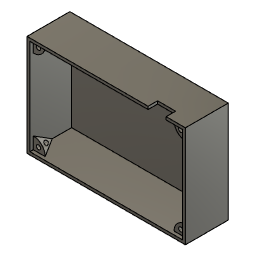
CR_R3 (Autodesk Fusion 360 design; units mm, degrees)
Autodesk Fusion 360 part; units mm, degrees
note: some values were not read from the file. Set by a fixed rule: which sketch regions a step uses.
sketch "Sketch1" plane through (0, 0, 0) normal (0, 0, 1) x (1, 0, 0)
  line L0 (1.5, 1.5) -> (82, 1.5)
  line L1 (82, 1.5) -> (82, 51.9)
  line L2 (82, 51.9) -> (1.5, 51.9)
  line L3 (1.5, 51.9) -> (1.5, 1.5)
  line L4 (83.5, 53.4) -> (0, 53.4)
  line L5 (0, 53.4) -> (0, 0)
  line L6 (0, 0) -> (83.5, 0)
  line L7 (83.5, 0) -> (83.5, 53.4)
  dimension "d6" = 50.4
  dimension "d8" = 1.5
  dimension "d112" = 80.5
  constraint horizontal L0
  constraint vertical L1
  constraint horizontal L2
  constraint vertical L3
  constraint coincident L5.end L6.start
  measures "d6" distance of L0.end L1.end
  measures "d112" distance of L1.end L2.end
extrude "Extrude2" add sketch "Sketch1" along normal blind 1 contours L0 L1 L2 L3
extrude "Extrude3" add sketch "Sketch1" along normal blind 23
sketch "Sketch4" plane through (0, 53.4, 0) normal (0, 1, 0) x (-1, 0, 0)
  line L0 (-83.5, 0) -> (0, 0)
  line L1 (0, 0) -> (0, 23)
  line L2 (0, 23) -> (-83.5, 23)
  line L3 (-83.5, 23) -> (-83.5, 0)
  line L4 (-63.8, 23) -> (-73.3, 23)
  line L5 (-63.8, 18) -> (-73.3, 18)
  line L6 (-73.3, 18) -> (-73.3, 23)
  line L7 (-63.8, 18) -> (-63.8, 23)
  dimension "d49" = 9.5
  dimension "d51" = 9.5
  dimension "d52" = 5
  dimension "d114" = 10.2
  constraint coincident L2 L4.start
  constraint coincident L2 L4.end
  constraint perpendicular L4 L6
  measures "d49" distance of L4.start L4.end
  measures "d51" distance of L5.start L5.end
  measures "d52" distance of L4 L5
  measures "d114" distance of L3 L6
extrude "Extrude8" cut sketch "Sketch4" against normal blind 1.5 contours L2 L4 L5 L6 L7
sketch "Sketch11" plane through (0, 51.9, 0) normal (0, -1, 0) x (1, 0, 0)
  line L0 (63.8, 23) -> (1.5, 23)
  line L1 (1.5, 23) -> (1.5, 1)
  line L2 (1.5, 1) -> (82, 1)
  line L3 (82, 1) -> (82, 23)
  line L4 (1.5, 21.2) -> (7.8, 21.2)
  line L5 (1.5, 21.2) -> (1.5, 11.2)
  line L6 (1.5, 11.2) -> (7.8, 21.2)
  line L7 (82, 21.2) -> (75.7, 21.2)
  line L8 (63.8, 18) -> (63.8, 23)
  line L9 (73.3, 18) -> (63.8, 18)
  line L10 (73.3, 23) -> (73.3, 18)
  line L11 (82, 23) -> (73.3, 23)
  line L12 (82, 21.2) -> (82, 11.2)
  line L13 (82, 11.2) -> (75.7, 21.2)
  dimension "d66" = 6.3
  dimension "d67" = 10
  dimension "d69" = 1.8
  dimension "d79" = 6.3
  dimension "d81" = 1.8
  dimension "d117" = 10
  constraint coincident L1 L4.start
  constraint perpendicular L1 L4
  constraint perpendicular L4 L5
  constraint coincident L3 L7.start
  constraint perpendicular L3 L7
  constraint perpendicular L7 L12
  measures "d66" distance of L4.start L4.end
  measures "d67" distance of L4.start L5.end
  measures "d69" distance of L0.end L4.start
  measures "d79" distance of L7.start L7.end
  measures "d81" distance of L3.end L7.start
  measures "d117" distance of L7.start L12.end
revolve "Revolve1" add sketch "Sketch11" angle 90 about axis through (1.5, 51.9, 21.2) along (0, 0, -1) contours L1 L4 L5 L6
sketch "Sketch12" plane through (0, 0, 21.2) normal (0, 0, 1) x (1, 0, 0)
  arc A0 (1.5, 45.6) -> (7.8, 51.9) centre (1.5, 51.9) ccw
  circle A1 centre (4.25, 49.4) radius 1.125
  line L0 (7.8, 51.9) -> (1.5, 51.9)
  line L1 (1.5, 51.9) -> (1.5, 45.6)
  dimension "d73" = 2.25
  dimension "d109" = 2.5
  dimension "d110" = 2.75
  measures "d73" diameter of A1
  measures "d109" distance of A1.centre L0
  measures "d110" distance of A1.centre L1
extrude "Extrude9" cut sketch "Sketch12" against normal blind 10 contours A1
revolve "Revolve2" add sketch "Sketch11" angle 90 about axis through (82, 51.9, 1) along (0, 0, 1) contours L3 L7 L12 L13
sketch "Sketch13" plane through (0, 0, 21.2) normal (0, 0, 1) x (1, 0, 0)
  line L0 (82, 45.6) -> (82, 51.9)
  circle A0 centre (79.25, 49.4) radius 1.125
  line L1 (82, 51.9) -> (75.7, 51.9)
  arc A1 (75.7, 51.9) -> (82, 45.6) centre (82, 51.9) ccw
  dimension "d86" = 2.25
  dimension "d87" = 2.75
  dimension "d118" = 2.5
  measures "d86" diameter of A0
  measures "d87" distance of L0 A0.centre
  measures "d118" distance of A0.centre L1
extrude "Extrude10" cut sketch "Sketch13" against normal blind 10 contours A0
sketch "Sketch14" plane through (0, 1.5, 0) normal (0, 1, 0) x (-1, 0, 0)
  line L0 (-82, 1) -> (-1.5, 1)
  line L1 (-1.5, 1) -> (-1.5, 23)
  line L2 (-1.5, 23) -> (-82, 23)
  line L3 (-82, 23) -> (-82, 1)
  line L4 (-82, 21.2) -> (-75.7, 21.2)
  line L5 (-75.7, 21.2) -> (-82, 11.2)
  line L6 (-82, 21.2) -> (-82, 11.2)
  line L7 (-1.5, 21.2) -> (-7.8, 21.2)
  line L8 (-7.8, 21.2) -> (-1.5, 11.2)
  line L9 (-1.5, 11.2) -> (-1.5, 21.2)
  line L10 (-63.8, 23) -> (0, 23)
  line L11 (-83.5, 23) -> (-73.3, 23)
  dimension "d91" = 1.8
  dimension "d92" = 10
  dimension "d93" = 6.3
  dimension "d95" = 6.3
  dimension "d96" = 10
  constraint coincident L3 L4.start
  constraint perpendicular L3 L4
  constraint coincident L3 L5.end
  constraint coincident L1 L7.start
  constraint perpendicular L1 L7
  constraint coincident L1 L8.end
  measures "d91" distance of L2.end L4.start
  measures "d92" distance of L4.start L5.end
  measures "d93" distance of L4.start L4.end
  measures "d95" distance of L7.start L7.end
  measures "d96" distance of L7.start L8.end
revolve "Revolve3" add sketch "Sketch14" angle 90 about axis through (82, 1.5, 23) along (0, 0, -1) contours L3 L4 L5 L6
revolve "Revolve4" add sketch "Sketch14" angle 90 about axis through (1.5, 1.5, 1) along (0, 0, 1) contours L1 L7 L8 L9
sketch "Sketch15" plane through (0, 0, 21.2) normal (0, 0, 1) x (1, 0, 0)
  line L0 (75.7, 1.5) -> (82, 1.5)
  line L1 (82, 1.5) -> (82, 7.8)
  arc A0 (82, 7.8) -> (75.7, 1.5) centre (82, 1.5) ccw
  circle A1 centre (79.25, 4) radius 1.125
  line L2 (82, 1.5) -> (75.7, 1.5)
  dimension "d99" = 2.25
  dimension "d100" = 2.5
  dimension "d101" = 2.75
  measures "d99" diameter of A1
  measures "d100" distance of A1.centre L2
  measures "d101" distance of L1 A1.centre
extrude "Extrude11" cut sketch "Sketch15" against normal blind 10 contours A1
sketch "Sketch16" plane through (0, 0, 21.2) normal (0, 0, 1) x (1, 0, 0)
  line L0 (1.5, 1.5) -> (7.8, 1.5)
  arc A0 (7.8, 1.5) -> (1.5, 7.8) centre (1.5, 1.5) ccw
  line L1 (1.5, 7.8) -> (1.5, 1.5)
  circle A1 centre (4.25, 4) radius 1.125
  line L2 (1.5, 1.5) -> (7.8, 1.5)
  dimension "d104" = 2.25
  dimension "d105" = 2.75
  dimension "d106" = 2.5
  measures "d104" diameter of A1
  measures "d105" distance of L1 A1.centre
  measures "d106" distance of A1.centre L2
extrude "Extrude12" cut sketch "Sketch16" against normal blind 10 contours A1
chamfer "Chamfer2" distance 0.4 angle 45 4 edges at (41.75, 0, 0) (83.5, 26.7, 0) (41.75, 53.4, 0) (0, 26.7, 0)
equation "width = 50.4 mm"
equation "length = 80.5 mm"
equation "height = 23 mm"
equation "thickness = 1.5 mm"
equation "d6 = width"
equation "d8 = thickness"
equation "mountDiamenter = 6 mm"
equation "mountHdistance = 68.83 mm"
equation "mountVdistance = 39.88 mm"
equation "d29 = height"
equation "holeDiameter = 2.25 mm"
equation "mountFillet = 3.5 mm"
equation "d66 = mountConeWidth"
equation "d67 = mountConeDepth"
equation "d69 = mountConeTopOffset"
equation "mountConeWidth = 6.3 mm"
equation "mountConeDepth = 10 mm"
equation "mountConeTopOffset = 1.8 mm"
equation "d73 = holeDiameter"
equation "d74 = -mountConeDepth"
equation "d79 = mountConeWidth"
equation "d81 = mountConeTopOffset"
equation "holeOffset_longSide = 2.5 mm"
equation "d86 = holeDiameter"
equation "d87 = holeOffset_shortSide"
equation "d89 = -mountConeDepth"
equation "d91 = mountConeTopOffset"
equation "d92 = mountConeDepth"
equation "d93 = mountConeWidth"
equation "d95 = mountConeWidth"
equation "d96 = mountConeDepth"
equation "d99 = holeDiameter"
equation "d100 = holeOffset_longSide"
equation "d101 = holeOffset_shortSide"
equation "d102 = -mountConeDepth"
equation "d104 = holeDiameter"
equation "d105 = holeOffset_shortSide"
equation "d106 = holeOffset_longSide"
equation "d107 = -mountConeDepth"
equation "d109 = holeOffset_longSide"
equation "d110 = holeOffset_shortSide"
equation "holeOffset_shortSide = 2.75 mm"
equation "d112 = length"
equation "d117 = mountConeDepth"
equation "d118 = holeOffset_longSide"
